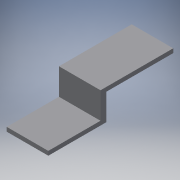
# Autodesk Inventor part: SyringeConnector
Saved by Autodesk Inventor 2018 (Build 220112000, 112)
## iProperties
Created: 2017-12-31
Part Number: SyringeConnector
Material: Generic
Document SubType Name: Modeling
Designer: reide
Density: 1 g/cm^3
Appearance: Default
Author: reide
Autodesk Inventor part; units mm, degrees
ref_plane "YZ Plane" through (0, 0, 0) normal (1, 0, 0) x (0, 1, 0)
sketch "Sketch1" plane through (0, 0, 0) normal (0, 0, 1) x (1, 0, 0)
  line L0 (4.2148, -12.63) -> (4.2148, -18.63) projected
  line L1 (0.6968, -12.63) -> (4.2148, -12.63) projected
  line L2 (0.6968, 12.63) -> (0.6968, -12.63) projected
  line L3 (16.6988, 12.63) -> (0.6968, 12.63) projected
  line L4 (16.6988, 17.202) -> (16.6988, 12.63) projected
  line L5 (21.6388, 17.202) -> (16.6988, 17.202) projected
  line L6 (21.6388, 12.63) -> (21.6388, 17.202) projected
  line L7 (23.7568, 12.63) -> (21.6388, 12.63) projected
  line L8 (23.7568, 18.63) -> (23.7568, 12.63) projected
  line L9 (-23.7568, 18.63) -> (23.7568, 18.63) projected
  line L10 (-23.7568, 12.63) -> (-23.7568, 18.63) projected
  line L11 (-21.6388, 12.63) -> (-23.7568, 12.63) projected
  line L12 (-21.6388, 17.202) -> (-21.6388, 12.63) projected
  line L13 (-16.6988, 17.202) -> (-21.6388, 17.202) projected
  line L14 (-16.6988, 12.63) -> (-16.6988, 17.202) projected
  line L15 (-0.6968, 12.63) -> (-16.6988, 12.63) projected
  line L16 (-0.6968, -12.63) -> (-0.6968, 12.63) projected
  line L17 (-4.2148, -12.63) -> (-0.6968, -12.63) projected
  line L18 (-4.2148, -18.63) -> (-4.2148, -12.63) projected
  line L19 (4.2148, -18.63) -> (-4.2148, -18.63) projected
  line L20 (0, 12.63) -> (10, 12.63)
  line L21 (10, 12.63) -> (-10, 12.63)
  line L22 (10, 12.63) -> (10, -22.37)
  line L23 (10, -22.37) -> (-10, -22.37)
  line L24 (-10, -22.37) -> (-10, 12.63)
  line L25 (-10, 12.63) -> (10, 12.63)
  line L26 (10, 12.63) -> (10, -22.37)
  point P0 (0, 0)
  dimension "d0" = 10
  dimension "d1" = 20
  dimension "d2" = 35
  constraints: 14 end point, 2 parallel, 2 perpendicular, 2 point on line, 1 horizontal
  measures "d0" distance of L20.start L20.end
  measures "d1" distance of L20.end L21.end
  measures "d2" distance of L20.end L22.end
extrude "Extrusion1" add sketch "Sketch1" along normal blind 2 contours L1 L2 L3 L22 L23 L24 L15 L16 L17 L18 L19 L0 | L0 L19 L18 L17 L16 L21 L20 L2 L1
sketch "Sketch2" plane through (0, 0, 0) normal (0, 0, -1) x (-1, 0, 0)
  line L0 (9.2308, -18.63) -> (23.7568, -18.63) projected
  line L1 (4.2148, -19.63) -> (-4.2148, -19.63) projected
  line L2 (10, 12.63) -> (10, -22.37) projected
  line L3 (-10, -22.37) -> (-10, 12.63) projected
  line L4 (10, -19.63) -> (-10, -19.63)
  line L5 (-10, -19.63) -> (-10, -22.37)
  line L6 (-10, -22.37) -> (10, -22.37)
  line L7 (10, -22.37) -> (10, -19.63)
  point P0 (0, 0)
  constraints: 8 end point, 2 parallel, 1 horizontal, 1 perpendicular, 1 point on line
ref_plane "Work Plane1" through (-27.5, -47.498, -12.7) normal (0, 0, 1) x (1, 0, 0)
extrude "Extrusion2" add sketch "Sketch2" along normal up to surface (12.7 mm away)
sketch "Sketch3" plane through (-10, -22.37, 2) normal (0, -1, 0) x (1, 0, 0)
  line L0 (0, -14.7) -> (0, 0) projected
  line L1 (0, -14.7) -> (0, -12.7)
  line L2 (20, -14.7) -> (20, 0) projected
  line L3 (0, -12.7) -> (20, -12.7)
  line L4 (20, -12.7) -> (20, -14.7)
  line L5 (20, -14.7) -> (0, -14.7)
  line L6 (0, -14.7) -> (0, -12.7)
  point P0 (10, -2)
  dimension "d7" = 2
  constraints: 10 end point, 2 parallel, 1 horizontal, 1 perpendicular, 1 point on line
  measures "d7" distance of L0.start L1.end
ref_plane "Work Plane2" through (-27.5, -47.498, -20.1034) normal (0, -1, 0) x (1, 0, 0)
extrude "Extrusion3" add sketch "Sketch3" along normal up to surface (25.128 mm away)
body "Solid1"
